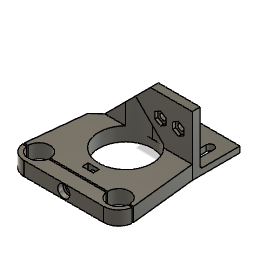
Laser Mounting Bracket v5 (Autodesk Fusion 360 design; units mm, degrees)
Autodesk Fusion 360 part; units mm, degrees
sketch "Sketch1" plane through (0, 0, 0) normal (0, 0, 1) x (1, 0, 0)
  line L0 (0, 0) -> (48, 0)
  line L1 (48, 0) -> (48, 27)
  line L2 (48, 27) -> (27, 27)
  line L3 (27, 27) -> (0, 0)
  line L4 (48, 0) -> (0, 0)
  line L5 (0, 0) -> (0, -3)
  line L6 (0, -3) -> (48, -3)
  line L7 (48, -3) -> (48, 0)
  circle A0 centre (41, 16) radius 1.65
  circle A1 centre (32, 16) radius 1.65
  line L8 (41, 12.7668) -> (43.8, 14.3834)
  line L9 (43.8, 14.3834) -> (43.8, 17.6166)
  line L10 (43.8, 17.6166) -> (41, 19.2332)
  line L11 (41, 19.2332) -> (38.2, 17.6166)
  line L12 (38.2, 17.6166) -> (38.2, 14.3834)
  line L13 (38.2, 14.3834) -> (41, 12.7668)
  line L14 (32, 12.7668) -> (34.8, 14.3834)
  line L15 (34.8, 14.3834) -> (34.8, 17.6166)
  line L16 (34.8, 17.6166) -> (32, 19.2332)
  line L17 (32, 19.2332) -> (29.2, 17.6166)
  line L18 (29.2, 17.6166) -> (29.2, 14.3834)
  line L19 (29.2, 14.3834) -> (32, 12.7668)
  point P0 (41, 16)
  point P1 (32, 16)
  dimension "d2" = 30
  dimension "d3" = 3
  dimension "d4" = 45
  dimension "d5" = 48
  dimension "d6" = 3.3
  dimension "d7" = 9
  dimension "d8" = 16
  dimension "d9" = 7
  dimension "d10" = 2.8
  constraint coincident L0.start L3.end
  constraint horizontal L0
  constraint perpendicular L0 L1
  constraint perpendicular L1 L2
  constraint horizontal L4
  constraint vertical L5
  constraint horizontal L6
  constraint vertical L7
  constraint coincident L0.start L5
  constraint equal A0 A1
  constraint horizontal P0 P1
  constraint coincident P0 A0.centre
  constraint vertical L8.start L10.end
  constraint coincident P1 A1.centre
  constraint equal L13 L19
  constraint vertical L14.start L16.end
  measures "d2" distance of L1.end L6.end
  measures "d3" distance of L0.start L5.end
  measures "d4" angle of L0 L3
  measures "d5" distance of L5.end L6.end
  measures "d6" diameter of A0
  measures "d7" distance of P0 P1
  measures "d8" vertical distance of L0.end P0
  measures "d9" horizontal distance of L0.end P0
  measures "d10" distance of P0 L13
extrude "Extrude1" add sketch "Sketch1" along normal blind 4 contours L0 L1 L2 L3 L4 | L0 L4 L5 L6 L7 | L8 L9 L10 L11 L12 L13 | L14 L15 L16 L17 L18 L19 makes body 1
extrude "Extrude2" cut sketch "Sketch1" against normal blind 1.5 from surface at 4 contours L8 L9 L10 L11 L12 L13 | L14 L15 L16 L17 L18 L19 bodies 1
extrude "Extrude3" add sketch "Sketch1" against normal blind 20 contours L0 L4 L5 L6 L7 bodies 1
sketch "Sketch2" plane through (0, 0, 0) normal (0, 1, 0) x (1, 0, 0)
  line L0 (9, 4) -> (9, 12)
  arc A0 (9, 12) -> (5, 12) centre (7, 12) ccw
  line L1 (5, 12) -> (5, 4)
  arc A1 (5, 4) -> (9, 4) centre (7, 4) ccw
  line L2 (7, 4) -> (7, 12) construction
  line L3 (39, 12) -> (39, 4)
  arc A2 (43, 12) -> (39, 12) centre (41, 12) ccw
  line L4 (43, 4) -> (43, 12)
  arc A3 (39, 4) -> (43, 4) centre (41, 4) ccw
  line L5 (41, 4) -> (41, 12) construction
  line L6 (0, 0) -> (0, 20) construction
  line L7 (48, 0) -> (48, 20) construction
  line L8 (0, 4) -> (7, 4) construction
  line L9 (41, 4) -> (48, 4) construction
  dimension "d18" = 4
  dimension "d19" = 4
  dimension "d20" = 8
  dimension "d21" = 34
  dimension "d22" = 4
  constraint tangent L0 A0
  constraint tangent A0 L1
  constraint parallel L0 L1
  constraint tangent L1 A1
  constraint tangent L0 A1
  constraint vertical L2
  constraint tangent A2 L4
  constraint tangent L3 A2
  constraint parallel L3 L4
  constraint tangent L3 A3
  constraint tangent L4 A3
  constraint coincident A3.centre L5.start
  constraint coincident A2.centre L5.end
  constraint vertical L5
  constraint equal L2 L5
  constraint horizontal A0.centre A2.centre
  constraint coincident L6 L8.start
  constraint coincident A1.centre L2.start
  constraint horizontal L8
  constraint coincident L7 L9.end
  constraint perpendicular L7 L9
  constraint equal L8 L9
  measures "d18" diameter of A0
  measures "d19" diameter of A2
  measures "d20" distance of A1.centre A0.centre
  measures "d21" distance of A1.centre A3.centre
  measures "d22" distance of L6.start L8.start
extrude "Extrude4" cut sketch "Sketch2" against normal through all bodies 1
fillet "Fillet1" radius 1 1 edges at (24, 0, 0) on bodies 1
sketch "Sketch3" plane through (0, 0, 0) normal (0, 1, 0) x (1, 0, 0)
  circle A0 centre (24, -13.5) radius 13.5
  line L0 (0, 0) -> (48, 0) construction
  line L1 (24, 0) -> (24, -13.5) construction
  line L2 (39, 12) -> (39, 4) construction
  dimension "d26" = 27
  dimension "d27" = 13.5
  constraint midpoint L0 L1.start
  constraint perpendicular L0 L1
  constraint coincident A0.centre L1.end
  measures "d26" diameter of A0
  measures "d27" distance of L1.start A0.centre
sketch "Sketch4" plane through (0, 0, 0) normal (0, 0, 1) x (1, 0, 0)
  line L0 (37.5, 0) -> (10.5, 0) construction
  line L1 (0, -3) -> (48, -3)
  line L2 (37.5, -3) -> (37.5, 1.5)
  line L3 (37.5, 1.5) -> (10.5, 28.5)
  line L4 (37.5, 1.5) -> (65.9887, 1.5) construction
  line L5 (10.5, -3) -> (10.5, 28.5)
  dimension "d29" = 4.5
  dimension "d30" = 135
  constraint coincident L1 L2.start
  constraint perpendicular L1 L2
  constraint coincident L0.start L2
  constraint horizontal L4
  constraint coincident L1 L5.start
  constraint perpendicular L1 L5
  constraint coincident L0.end L5
  constraint coincident L3.end L5.end
  measures "d29" distance of L2.start L2.end
  measures "d30" angle of L3 L4
extrude "Extrude5" add sketch "Sketch3" along normal blind 28.6 and the other way blind 3.1 separate body makes body 2
extrude "Extrude6" cut sketch "Sketch4" along normal through all and the other way through all keep common part bodies 2
sketch "Sketch5" plane through (0, 0, 0) normal (0, 1, 0) x (1, 0, 0)
  circle A0 centre (24, -13.5) radius 13.5
  circle A1 centre (24, -13.5) radius 13.5
  line L0 (32, -4) -> (29.2, -4)
  line L1 (29.2, -4) -> (32, -4)
  line L2 (32, -4) -> (34.8, -4)
  line L3 (34.8, -4) -> (32, -4)
  line L4 (41, -4) -> (38.2, -4)
  line L5 (38.2, -4) -> (41, -4)
  line L6 (41, -4) -> (43.8, -4)
  line L7 (43.8, -4) -> (41, -4)
  line L8 (48, -4) -> (27, -4)
  line L9 (27, -4) -> (0, -4)
  line L10 (0, -4) -> (48, -4)
  line L11 (44, -4) -> (4, -4) construction
  line L12 (4, -4) -> (4, -37) construction
  line L13 (4, -37) -> (44, -37) construction
  line L14 (44, -37) -> (44, -4) construction
  circle A2 centre (4, -37) radius 5.55
  circle A3 centre (44, -37) radius 5.55
  line L15 (44, -37) -> (24, -13.5) construction
  line L16 (24, -13.5) -> (4, -37) construction
  line L17 (7.8923, -33.0437) -> (7.2831, -32.5252) construction
  line L18 (24, -13.5) -> (24, -37) construction
  line L19 (0, -4) -> (-3.55, -37)
  line L20 (-3.55, -37) -> (-1.55, -37)
  line L21 (-3.55, -37) -> (-3.55, -37.8) construction
  line L22 (-3.55, -37.8) -> (-1.492, -37.8)
  arc A4 (-3.55, -37.8) -> (4, -44.5923) centre (4, -37) ccw
  line L23 (24, -37) -> (24, -44.5923) construction
  line L24 (24, -44.5923) -> (4, -44.5923)
  line L25 (9.55, -37) -> (38.45, -37)
  line L26 (9.492, -37.8) -> (38.508, -37.8)
  arc A5 (44, -44.5923) -> (51.55, -37.8) centre (44, -37) ccw
  line L27 (51.55, -37.8) -> (49.492, -37.8)
  line L28 (24, -44.5923) -> (44, -44.5923)
  line L29 (51.55, -37) -> (49.55, -37)
  line L30 (48, -4) -> (51.55, -37)
  line L31 (21.2, -29.5923) -> (26.8, -29.5923)
  line L32 (26.8, -29.5923) -> (26.8, -32.5923)
  line L33 (26.8, -32.5923) -> (21.2, -32.5923)
  line L34 (21.2, -32.5923) -> (21.2, -29.5923)
  point P0 (24, -4)
  point P1 (7.5877, -32.7844)
  point P2 (15.2504, -23.7808)
  point P3 (13.9542, -25.3039)
  point P4 (24, -29.5923)
  point P5 (24, -41.8923)
  dimension "d37" = 40
  dimension "d38" = 33
  dimension "d39" = 11.1
  dimension "d42" = 2
  dimension "d45" = 2
  dimension "d46" = 0.8
  dimension "d47" = 15
  dimension "d48" = 2.7
  dimension "d49" = 3
  dimension "d50" = 5.6
  constraint horizontal L11
  constraint vertical L12
  constraint horizontal L13
  constraint vertical L14
  constraint midpoint L11 P0
  constraint midpoint L10 P0
  constraint coincident L12.end L13.start
  constraint coincident L13.end L14.start
  constraint equal A2 A3
  constraint coincident A0.centre A1.centre
  constraint coincident A2 L17.end
  constraint coincident A2 L17.start
  constraint midpoint L17 P1
  constraint coincident L16 P1
  constraint coincident A1 P2
  constraint coincident L16 P2
  constraint coincident L16 P3
  constraint midpoint L13 L18.end
  constraint coincident L9.end L10.start
  constraint parallel L10 L20
  constraint collinear L13 L20
  constraint coincident A2 L20.end
  constraint perpendicular L20 L21
  constraint coincident A2 L22.end
  constraint perpendicular L21 L22
  constraint perpendicular L13 L23
  constraint horizontal L24
  constraint vertical L12.end A4.end
  constraint coincident A2 L25.start
  constraint coincident L13 L25.start
  constraint coincident A3 L25.end
  constraint coincident L13 L25.end
  constraint coincident A2 L26.start
  constraint coincident A3 L26.end
  constraint perpendicular L23 L26
  constraint collinear L22 L26
  constraint coincident L18 P4
  constraint coincident L23 P5
  constraint symmetric L9.end L23 L8.start
  constraint symmetric L19.end L23 L29.start
  constraint symmetric L20.end L23 L29.end
  constraint symmetric L21.end L23 A5.end
  constraint symmetric L22.end L23 L27.end
  constraint symmetric A4.end L23 A5.start
  constraint symmetric A4 L23 A5
  constraint symmetric L24.start L23 L28.start
  constraint horizontal L31
  constraint vertical L32
  constraint horizontal L33
  constraint vertical L34
  constraint midpoint P4 L31
  measures "d37" distance of L12.end L13.end
  measures "d38" distance of L11.start L13.end
  measures "d39" diameter of A2
  measures "d42" distance of P2 P3
  measures "d45" distance of L19.end L20.end
  measures "d46" distance of L19.end L21.end
  measures "d47" distance of L23.end P4
  measures "d48" distance of L23.end P5
  measures "d49" distance of L31.end L32.end
  measures "d50" distance of L31.start L31.end
combine "Combine1" operation cut target body 1 tool bodies 2
extrude "Extrude7" add sketch "Sketch5" along normal blind 7 from surface at -3 contours A0 A1 L2 L3 L4 L5 L6 L7 L8 L9 L10 A2 A3 L19 L20 L25 L29 L30 | A2 A3 L22 A4 L24 L26 A5 L27 L28 bodies 1 makes body 3 at (17.3333, 1.6667, 44.5923)
sketch "Sketch6" plane through (0.4254, 0, 0.0458) normal (-0.994263, 0, -0.106959) x (-0.106959, 0, 0.994263)
  line L0 (3.9771, -3) -> (37.1675, -3)
  line L1 (37.1675, -3) -> (37.1675, 4)
  line L2 (37.1675, 4) -> (3.9771, 4)
  line L3 (3.9771, 4) -> (3.9771, 0)
  line L4 (3.9771, 0) -> (3.9771, -3)
  line L5 (3.9771, 4) -> (7.9771, 4) construction
  point P0 (3.9771, 4)
  dimension "d54" = 4
  constraint coincident P0 L2.end
  constraint perpendicular L3 L5
  measures "d54" distance of P0 L5.end
ref_plane "WorkPlane1" through (4, 4, 4) normal (0.555595, -0.555595, 0.618569) x (0.707107, 0.707107, 0)
sketch "Sketch7" plane through (1.3747, -1.3747, 1.5305) normal (0.555595, -0.555595, 0.618569) x (0.707107, 0.707107, 0)
  line L0 (5.6569, 3.1429) -> (2.5259, 8.2045)
  line L1 (2.5259, 8.2045) -> (0, 3.1429)
  line L2 (0, 3.1429) -> (5.6569, 3.1429)
extrude "Extrude8" cut sketch "Sketch7" against normal up to surface (2.2224 mm away) bodies 1
sketch "Sketch8" plane through (0, 0, 44.5923) normal (0, 0, 1) x (1, 0, 0)
  line L0 (4, -3) -> (44, -3)
  line L1 (44, -3) -> (44, 4)
  line L2 (44, 4) -> (4, 4)
  line L3 (4, 4) -> (4, -3)
  line L4 (24, 4) -> (24, -3)
  point P0 (24, 0.5)
  constraint midpoint L2 L4.start
  constraint midpoint L0 L4.end
  constraint midpoint L4 P0
hole "Hole1" at (24, 0.5, 44.5923) direction (0, 0, -1) diameter 3.5 depth 20.593 tip angle 180 counterbore diameter 6.1 counterbore depth 2.6 bodies 1 3
equation "d30 = 180 deg - 45 deg"
